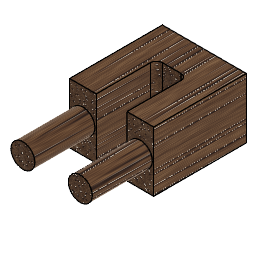
Prindere_Cadru (Autodesk Fusion 360 design; units mm, degrees)
part number: 2026-06-01-23-22-02-267
Autodesk Fusion 360 part; units mm, degrees
sketch "baza" plane through (0, 0, 0) normal (0, 0, 1) x (1, 0, 0)
  line L0 (1.275, 1.275) -> (-1.275, 1.275)
  line L1 (-1.275, 1.275) -> (-1.275, -1.275)
  line L2 (-1.275, -1.275) -> (1.275, -1.275)
  line L3 (1.275, -1.275) -> (1.275, 1.275)
  line L4 (1.275, 1.275) -> (-1.275, -1.275) construction
  line L5 (-1.275, 1.275) -> (1.275, -1.275) construction
  line L6 (3.5, 0) -> (3.5, -1.275)
  line L7 (-3.5, -1.275) -> (-3.5, 0)
  line L8 (-1.275, -1.275) -> (-3.5, -1.275)
  line L9 (1.275, -1.275) -> (3.5, -1.275)
  line L10 (3.5, 0) -> (3.5, 4)
  line L11 (3.5, 4) -> (-3.5, 4)
  line L12 (-3.5, 4) -> (-3.5, 0)
  line L13 (-1.275, -1.275) -> (-1.275, -3.725)
  line L14 (1.275, -1.275) -> (1.275, -3.725)
  line L15 (1.275, -3.725) -> (3.5, -3.725)
  line L16 (3.5, -3.725) -> (3.5, -1.275)
  line L17 (-3.5, -1.275) -> (-3.5, -3.725)
  line L18 (-3.5, -3.725) -> (-1.275, -3.725)
  line L19 (-1.275, 0.775) -> (1.275, 0.775)
  dimension "d1" = 2.55
  dimension "d4" = 7
  dimension "d11" = 7
  dimension "d12" = 4
  dimension "d16" = 1.275
  dimension "d17" = 2.45
  dimension "d18" = 0.5
  constraint horizontal L0
  constraint perpendicular L0 L1
  constraint parallel L0 L2
  constraint parallel L1 L3
  constraint coincident L4 origin
  constraint coincident L5 origin
  constraint vertical L6
  constraint vertical L7
  constraint perpendicular L7 L8
  constraint perpendicular L6 L9
  constraint vertical L10
  constraint horizontal L11
  constraint vertical L12
  constraint perpendicular L2 L13
  constraint perpendicular L2 L14
  constraint perpendicular L6 L15
  constraint perpendicular L9 L16
  constraint perpendicular L8 L17
  constraint perpendicular L13 L18
  constraint coincident L1 L19.start
  constraint coincident L3 L19.end
  constraint perpendicular L3 L19
  measures "d1" distance of L1.end L2.end
  measures "d4" distance of L7.end L6.start
  measures "d11" distance of L7.end L6.start
  measures "d12" distance of L7.end L11.end
  measures "d16" distance of L2 origin
  measures "d17" distance of L1.end L13.end
  measures "d18" distance of L0 L19
extrude "Extrude1" add sketch "baza" along normal blind 5 contours L0 L1 L3 L6 L7 L8 L9 L10 L11 L12 | L9 L14 L15 L16 | L8 L13 L17 L18
sketch "dinti" plane through (0, -3.725, 0) normal (0, -1, 0) x (1, 0, 0)
  line L0 (-3.5, 0) -> (-1.275, 0)
  line L1 (-1.275, 0) -> (-1.275, 5)
  line L2 (-1.275, 5) -> (-3.5, 5)
  line L3 (-3.5, 5) -> (-3.5, 0)
  line L4 (-2.3875, 5) -> (-2.3875, 0) construction
  circle A0 centre (-2.3875, 2.5) radius 1
  line L5 (-1.275, 0) -> (1.275, 0) construction
  line L6 (1.275, 0) -> (1.275, 5) construction
  line L7 (1.275, 5) -> (-1.275, 5) construction
  line L8 (-1.275, 5) -> (-1.275, 0) construction
  line L9 (0, 5) -> (0, 0) construction
  circle A1 centre (2.3875, 2.5) radius 1
  line L10 (-3.5, 0) -> (-1.275, 0)
  line L11 (-1.275, 0) -> (-1.275, 5)
  line L12 (-1.275, 5) -> (-3.5, 5)
  line L13 (-3.5, 5) -> (-3.5, 0)
  dimension "d8" = 2
  constraint midpoint L2 L4.start
  constraint midpoint L0 L4.end
  constraint midpoint L4 A0.centre
  constraint midpoint L7 L9.start
  constraint coincident L9.end origin
  constraint symmetric A0 L9 A1
  measures "d8" diameter of A0
extrude "Extrude2" add sketch "dinti" along normal blind 5 contours A0 | A1
fillet "Fillet1" radius 0.5 2 edges at (1.275, 1.275, 2.5) (-1.275, 1.275, 2.5)
equation "d17 = 3.725 mm - 1.275 mm"
named bodies: "Prindere"
